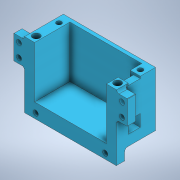
# Autodesk Inventor part: мотор_плеча_1v2
Saved by Autodesk Inventor 2022 (Build 260153000, 153)
## iProperties
Created: 2022-12-03
Part Number: мотор_плеча_1v2
Material: Типовые
Document SubType Name: Modeling
Designer: Папа
Density: 1 g/cm^3
Appearance: По умолчанию
Author: Папа
Autodesk Inventor part; units mm, degrees
sketch "Эскиз1" plane through (0, 0, 0) normal (0, 1, 0) x (-1, 0, 0)
  line L0 (0, 0) -> (-60, 0)
  line L1 (-60, 0) -> (-60, -29.5)
  line L2 (-60, -29.5) -> (0, -29.5)
  line L3 (0, -29.5) -> (0, 0)
  line L4 (-68.5, 3) -> (8.5, 3)
  line L5 (8.5, 3) -> (8.5, -32.5)
  line L6 (8.5, -32.5) -> (-68.5, -32.5)
  line L7 (-68.5, -32.5) -> (-68.5, 3)
  line L8 (-68.5, 3) -> (8.5, -32.5) construction
  line L9 (8.5, 3) -> (-68.5, -32.5) construction
  line L10 (0, -29.5) -> (-60, 0) construction
  line L11 (0, 0) -> (-60, -29.5) construction
  line L12 (8.5, 0) -> (-68.5, 0)
  point P0 (-30, -14.75)
  point P1 (-30, -14.75)
  point P2 (0, 0)
  dimension "d0" = 29.5
  dimension "d1" = 60
  dimension "d3" = 3
  dimension "d77" = 77
  constraints: 26 end point, 4 midpoint, 4 parallel, 3 point on line, 2 horizontal, 2 perpendicular, 1 collinear
  measures "d0" distance of L2.end L0.start
  measures "d1" distance of L1.end L2.end
  measures "d3" distance between parallel lines of L6 L2
  measures "d77" distance between parallel lines of L7 L5
extrude "Выдавливание1" add sketch "Эскиз1" along normal blind 43 contours L12 L5 L6 L7 L1 L2 L3
sketch "Эскиз2" plane through (0, 0, 0) normal (0, -1, 0) x (1, 0, 0)
  line L0 (68.5, 0) -> (68.5, -32.5) projected
  line L1 (-8.5, -32.5) -> (-8.5, 0) projected
  line L2 (68.5, 0) -> (-8.5, 0)
  line L3 (-8.5, 0) -> (-8.5, -32.5)
  line L4 (-8.5, -32.5) -> (68.5, -32.5)
  line L5 (68.5, -32.5) -> (68.5, 0)
  point P0 (0, 0)
  point P1 (-8.5, 0)
  constraints: 8 end point, 2 parallel, 1 horizontal, 1 perpendicular
extrude "Выдавливание2" add sketch "Эскиз2" along normal blind 3
sketch "Эскиз3" plane through (0, 43, 0) normal (0, 1, 0) x (1, 0, 0)
  circle A0 centre (-4, 5.35) radius 2.1
  circle A1 centre (-4, 24.35) radius 2.1
  circle A2 centre (64, 24.35) radius 2.1
  circle A3 centre (64, 5.35) radius 2.1
  line L0 (60, 29.5) -> (60, 0) construction
  line L1 (0, 0) -> (0, 29.5) construction
  line L2 (60, 29.5) -> (0, 29.5) construction
  line L3 (0, 29.5) -> (0, 0.2) construction
  line L4 (0, 0.2) -> (60, 0.2) construction
  line L5 (60, 0.2) -> (60, 29.5) construction
  line L6 (0, 0) -> (60, 0) construction
  line L7 (60, 0) -> (60, 0.2) construction
  line L8 (60, 0.2) -> (0, 0.2) construction
  line L9 (0, 0.2) -> (0, 0) construction
  line L10 (0, 0.2) -> (60, 29.5) construction
  line L11 (60, 0.2) -> (0, 29.5) construction
  line L12 (-4, 5.35) -> (64, 5.35) construction
  line L13 (64, 5.35) -> (64, 24.35) construction
  line L14 (64, 24.35) -> (-4, 24.35) construction
  line L15 (-4, 24.35) -> (-4, 5.35) construction
  line L16 (-4, 5.35) -> (64, 24.35) construction
  line L17 (-4, 24.35) -> (64, 5.35) construction
  point P0 (30, 14.85)
  dimension "d8" = 4.2
  dimension "d70" = 0.2
  dimension "d72" = 19
  dimension "d73" = 68
  constraints: 32 end point, 6 parallel, 4 centre point, 3 equal radius, 3 horizontal, 3 perpendicular, 2 coincident, 2 midpoint, 1 point on line
  measures "d8" diameter of A0
  measures "d70" distance between parallel lines of L4 L6
  measures "d72" distance of L13.end A3.centre
  measures "d73" distance of L13.end L14.end
extrude "Выдавливание3" cut sketch "Эскиз3" against normal blind 30
ref_plane "РабПлоскость1" through (0, 18, 0) normal (0, 1, 0) x (1, 0, 0)
ref_plane "РабПлоскость2" through (0, 20, 0) normal (0, -1, 0) x (1, 0, 0)
sketch "Эскиз8" plane through (60, 43, 0) normal (0, 0, 1) x (1, 0, 0)
  line L0 (0, -43) -> (-60, -43) projected
  line L1 (-68.5, -46) -> (8.5, -46) projected
  line L2 (-56.0151, -43.2389) -> (-56.0151, -54.3) construction
  line L3 (-59, -46) -> (-59, -55)
  line L4 (-54.5, -46) -> (-63.5, -46)
  line L5 (-63.5, -46) -> (-63.5, -55)
  line L6 (-63.5, -55) -> (-54.5, -55)
  line L7 (-54.5, -55) -> (-54.5, -46)
  line L8 (-54.5, -46) -> (-63.5, -55) construction
  line L9 (-63.5, -46) -> (-54.5, -55) construction
  circle A0 centre (-59, -50.5) radius 2.1
  line L10 (-68.5, -46) -> (-68.5, 0) projected
  line L11 (-68.5, -46) -> (-68.5, 0) projected
  line L12 (-68.5, -2) -> (-77.5, -2)
  line L13 (-77.5, -2) -> (-77.5, -22)
  line L14 (-77.5, -22) -> (-68.5, -22)
  line L15 (-68.5, -22) -> (-68.5, -2)
  line L16 (-68.5, -2) -> (-77.5, -11) construction
  line L17 (-68.5, -22) -> (-77.5, -13) construction
  circle A1 centre (-73, -6.5) radius 2.1
  circle A2 centre (-73, -17.5) radius 2.1
  line L18 (8.5, -46) -> (-68.5, -46) projected
  point P0 (-68.025, -27.3)
  dimension "d42" = 8.3
  dimension "d44" = 9
  dimension "d45" = 9
  dimension "d46" = 4.2
  dimension "d78" = 5
  dimension "d79" = 9
  dimension "d80" = 2
  dimension "d81" = 20
  dimension "d82" = 9
  dimension "d83" = 9
  dimension "d84" = 4.2
  constraints: 28 end point, 5 midpoint, 4 parallel, 3 centre point, 3 point on line, 2 horizontal, 2 perpendicular, 2 vertical, 1 coincident, 1 collinear, 1 equal radius, 3 other
  measures "d42" distance from line of L2.end L1
  measures "d44" distance of L3.start L3.end
  measures "d45" distance between parallel lines of L7 L5
  measures "d46" diameter of A0
  measures "d79" distance of L12.start L12.end
  measures "d80" distance from line of L12 point (-68.5, 0)
  measures "d81" distance of L12.end L13.end
  measures "d82" distance of L12.end L16.end
  measures "d83" distance of L13.end L17.end
  measures "d84" diameter of A2
extrude "Выдавливание8" add sketch "Эскиз8" against normal blind 7 contours L1 L3 A0 L6 L5 | L1 L7 L6 L3 A0 | L14 L13 L12 L10
sketch "Эскиз9" plane through (60, 43, -7) normal (0, 0, -1) x (-1, 0, 0)
  circle A0 centre (59, -50.5) radius 2.1 projected
  line L0 (59, -54.6281) -> (55.425, -52.564)
  line L1 (55.425, -52.564) -> (55.425, -48.436)
  line L2 (55.425, -48.436) -> (59, -46.3719)
  line L3 (59, -46.3719) -> (62.575, -48.436)
  line L4 (62.575, -48.436) -> (62.575, -52.564)
  line L5 (62.575, -52.564) -> (59, -54.6281)
  circle A1 centre (73, -17.5) radius 2.1 projected
  line L6 (77.1281, -17.5) -> (75.064, -21.075)
  line L7 (75.064, -21.075) -> (70.936, -21.075)
  line L8 (70.936, -21.075) -> (68.8719, -17.5)
  line L9 (68.8719, -17.5) -> (70.936, -13.925)
  line L10 (70.936, -13.925) -> (75.064, -13.925)
  line L11 (75.064, -13.925) -> (77.1281, -17.5)
  circle A2 centre (73, -6.5) radius 2.1 projected
  line L12 (77.1281, -6.5) -> (75.064, -10.075)
  line L13 (75.064, -10.075) -> (70.936, -10.075)
  line L14 (70.936, -10.075) -> (68.8719, -6.5)
  line L15 (68.8719, -6.5) -> (70.936, -2.925)
  line L16 (70.936, -2.925) -> (75.064, -2.925)
  line L17 (75.064, -2.925) -> (77.1281, -6.5)
  point P0 (60, -43)
  dimension "d49" = 7.15
  constraints: 36 end point, 3 coincident, 2 equal length, 2 horizontal, 1 vertical, 39 other
  measures "d49" distance between parallel lines of L1 L4
extrude "Выдавливание9" cut sketch "Эскиз9" against normal blind 3 contours L0 L1 L2 L3 L4 L5 | L6 L7 L8 L9 L10 L11 | A2 | L12 L13 L14 L15 L16 L17
sketch "Эскиз10" plane through (0, 43, 0) normal (0, 1, 0) x (1, 0, 0)
  line L0 (60, 0) -> (68.5, 0) projected
  line L1 (68.5, 32.5) -> (-8.5, 32.5) projected
  line L2 (68.5, 0) -> (-8.5, 0)
  line L3 (-8.5, 0) -> (-8.5, 32.5)
  line L4 (-8.5, 32.5) -> (68.5, 32.5)
  line L5 (68.5, 32.5) -> (68.5, 0)
  line L6 (0, 0) -> (0, 29.5) projected
  line L7 (60, 29.5) -> (60, 0) projected
  line L8 (0, 29.5) -> (60, 29.5)
  line L9 (60, 29.5) -> (60, 0)
  line L10 (60, 0) -> (0, 0)
  line L11 (0, 0) -> (0, 29.5)
  circle A0 centre (64, 24.35) radius 2.1 projected
  circle A1 centre (64, 24.35) radius 2.05
  circle A2 centre (63.55, 5.0621) radius 2.05
  circle A3 centre (-4, 5.35) radius 2.1 projected
  circle A4 centre (-4, 5.35) radius 2.05
  circle A5 centre (-4.45, 24.05) radius 2.05
  point P0 (68.5, 32.5)
  constraints: 16 end point, 4 centre point, 4 parallel, 2 coincident, 2 horizontal, 2 perpendicular
extrude "Выдавливание10" add sketch "Эскиз10" along normal blind 7 contours L7 L8 L6 L2 L3 L1 L5 L0
sketch "Эскиз15" plane through (0, 50, 0) normal (0, 1, 0) x (1, 0, 0)
  line L0 (-39.922, -21.3625) -> (76.3615, -21.3625)
  line L1 (76.3615, -21.3625) -> (76.3615, 38.0109)
  line L2 (76.3615, 38.0109) -> (-39.922, 38.0109)
  line L3 (-39.922, 38.0109) -> (-39.922, -21.3625)
  point P0 (0, 0)
  constraints: 8 end point, 2 parallel, 1 horizontal, 1 perpendicular
extrude "Выдавливание13" cut sketch "Эскиз15" against normal up to surface (7 mm away)
ref_plane "РабПлоскость6" through (30, -3, 0) normal (1, 0, 0) x (0, 0, -1)
mirror "Зеркальное отражение5" about plane through (30, -3, 0) normal (1, 0, 0) of "Выдавливание8", "Выдавливание9"
sketch "Эскиз17" plane through (54.5, -12, 0) normal (-1, 0, 0) x (0, 0, 1)
  line L0 (0, 9) -> (0, 0) projected
  line L1 (0, 0) -> (-7, 0) projected
  line L2 (-7, 0) -> (-7, 9) projected
  line L3 (0, 9) -> (-7, 9) projected
  point P0 (0, 12)
extrude "Выдавливание14" add sketch "Эскиз17" along normal up to surface (49.925 mm away)
sketch "Эскиз18" plane through (-3.5, -12, 0) normal (-1, 0, 0) x (0, 0, 1)
  line L0 (0, 9) -> (0, 0) projected
  line L1 (-7, 9) -> (0, 9) projected
  line L2 (-7, 0) -> (-7, 9) projected
  line L3 (0, 0) -> (-7, 0) projected
  point P0 (0, 12)
extrude "Выдавливание15" add sketch "Эскиз18" along normal up to surface (5 mm away)
sketch "Эскиз19" plane through (63.5, -12, 0) normal (1, 0, 0) x (0, 0, -1)
  line L0 (0, 9) -> (0, 0) projected
  line L1 (0, 0) -> (7, 0) projected
  line L2 (7, 0) -> (7, 9) projected
  line L3 (0, 9) -> (7, 9) projected
  point P0 (0, 12)
extrude "Выдавливание16" add sketch "Эскиз19" along normal up to surface (5 mm away)
fillet "Сопряжение18" radius 2 3 edges at (30, -3, -7) (-8.5, 31, -7) (68.5, 31, -7)
fillet "Сопряжение19" radius 2 4 edges at (-8.5, 21, -4.5) (-8.5, 41, -4.5) (68.5, 41, -4.5) (68.5, 21, -4.5)
fillet "Сопряжение20" radius 0.3 23 edges at (77.5, 41, -3.5) (70.4999, 41, -7) (74, 41, -7) (77.5, 31, -7) (77.5, 21, -3.5) (70.4999, 21, -7) (74, 21, -7) (68.5, -3.5858, -7.5858) (68.5, -3, -20.75) (68.5, -8.5, -7) (30, -12, -7) (-8.5, -3.5858, -7.5858) (-8.5, -3, -20.75) (-8.5, -8.5, -7) (-8.5, -12, -3.5) (68.5, -12, -3.5) (-17.5, 21, -3.5) (-10.4999, 21, -7) (-14, 21, -7) (-17.5, 31, -7) (-10.4999, 41, -7) (-14, 41, -7) (-17.5, 41, -3.5)
sketch "Эскиз20" plane through (60, 43, -29.5) normal (-1, 0, 0) x (0, 0, 1)
  line L0 (7.25, 0) -> (3.05, 0) projected
  line L1 (22.05, 0) -> (26.25, 0) projected
  line L2 (7.25, 0) -> (22.05, 0)
  line L3 (22.05, 0) -> (22.05, -30) projected
  line L4 (9.75, 37) -> (9.75, -37)
  line L5 (9.75, -37) -> (19.75, -37)
  line L6 (19.75, -37) -> (19.75, 37)
  line L7 (19.75, 37) -> (9.75, 37)
  line L8 (29.5, 0) -> (0, 0) projected
  line L9 (9.75, 37) -> (19.75, -37) construction
  line L10 (9.75, -37) -> (19.75, 37) construction
  point P0 (29.5, -43)
  point P1 (14.75, 0)
  dimension "d101" = 10
  dimension "d102" = 37
  constraints: 14 end point, 3 midpoint, 3 perpendicular, 2 parallel
  measures "d101" distance of L4.end L5.end
  measures "d102" distance from line of L5 point (14.75, 0)
extrude "Выдавливание17" cut sketch "Эскиз20" against normal blind 3
sketch "Эскиз21" plane through (63, 43, -29.5) normal (-1, 0, 0) x (0, 0, 1)
  line L0 (9.75, -37) -> (9.75, 0) projected
  line L1 (19.75, 0) -> (19.75, -37) projected
  line L2 (9.75, -37) -> (9.75, 0) projected
  line L3 (19.75, 0) -> (19.75, -37) projected
  line L4 (9.75, 0) -> (19.75, 0)
  line L5 (19.75, 0) -> (19.75, -1.75)
  line L6 (19.75, -1.75) -> (9.75, -1.75)
  line L7 (9.75, -1.75) -> (9.75, 0)
  point P0 (29.5, -43)
  dimension "d105" = 1.75
  constraints: 8 end point, 2 parallel, 1 horizontal, 1 perpendicular, 1 point on line
  measures "d105" distance between parallel lines of L4 L6
extrude "Выдавливание18" cut sketch "Эскиз21" against normal blind 100
sketch "Эскиз23" plane through (64, 13, -24.35) normal (0, 1, 0) x (1, 0, 0)
  circle A0 centre (-68, 0) radius 2.1 projected
  circle A1 centre (0, 0) radius 2.1 projected
  point P0 (-64, -24.35)
extrude "Выдавливание20" cut sketch "Эскиз23" against normal blind 100
sketch "Эскиз24" plane through (0, -3, 0) normal (0, -1, 0) x (1, 0, 0)
  circle A0 centre (-4, -24.35) radius 2.1 projected
  circle A1 centre (-4, -24.35) radius 3
  circle A2 centre (64, -24.35) radius 2.1 projected
  circle A3 centre (64, -24.35) radius 3
  point P0 (0, 0)
  dimension "d113" = 6
  dimension "d114" = 6
  constraints: 2 centre point, 2 coincident
  measures "d113" diameter of A1
  measures "d114" diameter of A3
extrude "Выдавливание21" cut sketch "Эскиз24" against normal blind 8.2 contours A0 | A1 | A2 | A3
sketch "Эскиз25" plane through (0, 43, 0) normal (0, 1, 0) x (1, 0, 0)
  circle A0 centre (64, 5.35) radius 2.1 projected
  circle A1 centre (64, 5.35) radius 3
  circle A2 centre (-4, 5.35) radius 2.1 projected
  circle A3 centre (-4, 5.35) radius 3
  point P0 (0, 0)
  dimension "d117" = 6
  dimension "d118" = 6
  constraints: 2 centre point, 2 coincident
  measures "d117" diameter of A3
  measures "d118" diameter of A1
extrude "Выдавливание22" cut sketch "Эскиз25" against normal blind 8.2 contours A0 | A1 | A2 | A3
sketch "Эскиз26" plane through (63, 43, -29.5) normal (-1, 0, 0) x (0, 0, 1)
  line L0 (19.75, -1.75) -> (9.75, -1.75) projected
  line L1 (9.75, -37) -> (9.75, -1.75) projected
  line L2 (19.75, -37) -> (9.75, -37) projected
  line L3 (19.75, -1.75) -> (19.75, -37) projected
  line L4 (19.75, -37) -> (9.75, -37) projected
  line L5 (9.75, -37) -> (19.75, -37)
  line L6 (19.75, -37) -> (19.75, -27)
  line L7 (19.75, -27) -> (9.75, -27)
  line L8 (9.75, -27) -> (9.75, -37)
  point P0 (29.5, -43)
  dimension "d121" = 10
  constraints: 8 end point, 2 parallel, 1 horizontal, 1 perpendicular, 1 point on line
  measures "d121" distance between parallel lines of L7 L2
extrude "Выдавливание23" cut sketch "Эскиз26" against normal blind 10 contours L3 L2 L1 L7
